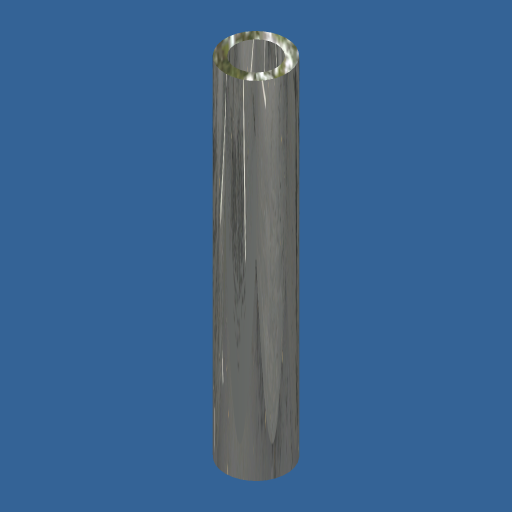
# Autodesk Inventor part: ArmSpindleTube
Saved by Autodesk Inventor 2023 (Build 270158030, 158C)
## iProperties
Created: 2023-02-27
Part Number: ArmSpindleTube
Material: Aluminum 6061
Document SubType Name: Modeling
Designer: kumpu
Density: 2.7 g/cm^3
Appearance: Aluminum - Flat
Author: kumpu
Autodesk Inventor part; units mm, degrees
ref_plane "YZ Plane" through (0, 0, 0) normal (1, 0, 0) x (0, 1, 0)
ref_plane "XZ Plane" through (0, 0, 0) normal (0, 1, 0) x (-1, 0, 0)
ref_plane "XY Plane" through (0, 0, 0) normal (0, 0, 1) x (1, 0, 0)
sketch "Sketch1" plane through (0, 0, 0) normal (1, 0, 0) x (0, 1, 0)
  line L0 (107.95, -12.7) -> (-107.95, -12.7)
  line L1 (-107.95, -12.7) -> (-107.95, -19.05)
  line L2 (-107.95, -19.05) -> (107.95, -19.05)
  line L3 (107.95, -19.05) -> (107.95, -12.7)
  line L4 (107.95, 0) -> (-107.95, 0) construction
  point P0 (0, 0)
  point P1 (0, 0)
  dimension "d0" = 215.9
  dimension "d1" = 6.35
  dimension "d2" = 38.1
  constraints: 10 end point, 2 horizontal, 2 parallel, 2 point on line, 1 coincident, 1 midpoint, 1 perpendicular
  measures "d0" distance of L1.end L2.end
  measures "d1" distance of L2.end L0.start
  measures "d2" diameter of L2 L4
revolve "Revolution1" add sketch "Sketch1" angle 360 about axis through (0, 107.95, 0) along (0, -1, 0)
body "Solid1"
